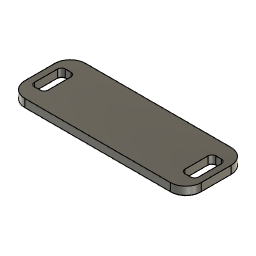
magnet spacer v1 (Autodesk Fusion 360 design; units mm, degrees)
Autodesk Fusion 360 part; units mm, degrees
sketch "Sketch1" plane through (0, 0, 0) normal (0, 0, 1) x (1, 0, 0)
  line L0 (4, 0) -> (41.72, 0)
  line L1 (45.72, 4) -> (45.72, 11.75)
  line L2 (41.72, 15.75) -> (4, 15.75)
  line L3 (0, 11.75) -> (0, 0)
  line L4 (0, 7.8501) -> (45.72, 7.875)
  line L5 (0, 15.75) -> (3.36, 15.75)
  line L6 (3.36, 15.75) -> (3.36, 0)
  line L7 (3.36, 0) -> (0, 0)
  line L8 (0, 4) -> (0, 15.75)
  line L9 (45.72, 15.75) -> (42.36, 15.75)
  line L10 (42.36, 15.75) -> (42.36, 0)
  line L11 (42.36, 0) -> (45.72, 0)
  line L12 (45.72, 0) -> (45.72, 15.75)
  line L13 (4.11, 11.875) -> (2.61, 11.875)
  line L14 (1.61, 10.875) -> (1.61, 4.875)
  line L15 (2.61, 3.875) -> (4.11, 3.875)
  line L16 (5.11, 4.875) -> (5.11, 10.875)
  line L17 (5.11, 11.875) -> (1.61, 3.875) construction
  line L18 (1.61, 11.875) -> (5.11, 3.875) construction
  line L19 (41.61, 11.875) -> (43.11, 11.875)
  line L20 (44.11, 10.875) -> (44.11, 4.875)
  line L21 (43.11, 3.875) -> (41.61, 3.875)
  line L22 (40.61, 4.875) -> (40.61, 10.875)
  line L23 (40.61, 11.875) -> (44.11, 3.875) construction
  line L24 (44.11, 11.875) -> (40.61, 3.875) construction
  arc A0 (5.11, 10.875) -> (4.11, 11.875) centre (4.11, 10.875) ccw
  arc A1 (2.61, 11.875) -> (1.61, 10.875) centre (2.61, 10.875) ccw
  arc A2 (1.61, 4.875) -> (2.61, 3.875) centre (2.61, 4.875) ccw
  arc A3 (4.11, 3.875) -> (5.11, 4.875) centre (4.11, 4.875) ccw
  arc A4 (41.61, 11.875) -> (40.61, 10.875) centre (41.61, 10.875) ccw
  arc A5 (40.61, 4.875) -> (41.61, 3.875) centre (41.61, 4.875) ccw
  arc A6 (43.11, 3.875) -> (44.11, 4.875) centre (43.11, 4.875) ccw
  arc A7 (44.11, 10.875) -> (43.11, 11.875) centre (43.11, 10.875) ccw
  arc A8 (45.72, 11.75) -> (41.72, 15.75) centre (41.72, 11.75) ccw
  arc A9 (0, 4) -> (4, 0) centre (4, 4) ccw
  arc A10 (4, 15.75) -> (0, 11.75) centre (4, 11.75) ccw
  arc A11 (41.72, 0) -> (45.72, 4) centre (41.72, 4) ccw
  point P0 (45.72, 0)
  point P1 (3.36, 7.875)
  point P2 (42.36, 7.875)
  dimension "d1" = 45.72
  dimension "d2" = 15.75
  dimension "d5" = 3.36
  dimension "d6" = 15.75
  dimension "d7" = 3.36
  dimension "d8" = 15.75
  dimension "d9" = 3.5
  dimension "d10" = 8
  dimension "d11" = 3.5
  dimension "d12" = 8
  dimension "d13" = 1
  dimension "d14" = 1
  dimension "d15" = 4
  dimension "d16" = 4
  constraint horizontal L0
  constraint vertical L1
  constraint horizontal L2
  constraint vertical L3
  constraint coincident L3.end L7.end
  constraint coincident L3 L4.start
  constraint horizontal L5
  constraint vertical L6
  constraint horizontal L7
  constraint vertical L8
  constraint horizontal L9
  constraint vertical L10
  constraint horizontal L11
  constraint vertical L12
  constraint horizontal L13
  constraint perpendicular L13 L14
  constraint parallel L13 L15
  constraint parallel L14 L16
  constraint coincident L17 P1
  constraint coincident L18 P1
  constraint midpoint L6 P1
  constraint horizontal L19
  constraint perpendicular L19 L20
  constraint parallel L19 L21
  constraint parallel L20 L22
  constraint coincident L23 P2
  constraint coincident L24 P2
  constraint midpoint L10 P2
  constraint coincident L17.start L13
  constraint coincident L17.start L16
  constraint tangent L13 A0
  constraint tangent L16 A0
  constraint coincident L18.start L13
  constraint coincident L18.start L14
  constraint tangent L13 A1
  constraint tangent L14 A1
  constraint equal A0 A1
  constraint coincident L17.end L14
  constraint coincident L17.end L15
  constraint tangent L14 A2
  constraint tangent L15 A2
  constraint equal A0 A2
  constraint coincident L18.end L15
  constraint coincident L18.end L16
  constraint tangent L15 A3
  constraint tangent L16 A3
  constraint equal A0 A3
  constraint coincident L23.start L19
  constraint coincident L23.start L22
  constraint tangent L19 A4
  constraint tangent L22 A4
  constraint equal A0 A4
  constraint coincident L24.end L22
  constraint coincident L24.end L21
  constraint tangent L22 A5
  constraint tangent L21 A5
  constraint equal A0 A5
  constraint coincident L23.end L21
  constraint coincident L23.end L20
  constraint tangent L21 A6
  constraint tangent L20 A6
  constraint equal A0 A6
  constraint coincident L24.start L20
  constraint coincident L24.start L19
  constraint tangent L20 A7
  constraint tangent L19 A7
  constraint coincident L1 L4.end
  constraint coincident L9.start L2
  constraint coincident L9.start L1
  constraint tangent L2 A8
  constraint tangent L1 A8
  constraint coincident L3.end L8
  constraint coincident L3.end L0
  constraint tangent L8 A9
  constraint tangent L0 A9
  constraint coincident L5.start L2
  constraint coincident L5.start L3
  constraint tangent L2 A10
  constraint tangent L3 A10
  constraint equal A9 A10
  constraint coincident P0 L0
  constraint coincident P0 L1
  constraint tangent L0 A11
  constraint tangent L1 A11
  constraint equal A9 A11
  measures "d1" distance of L3.end P0
  measures "d2" distance of L3.end L5.start
  measures "d5" distance of L5.start L5.end
  measures "d6" distance of L5.start L3.end
  measures "d7" distance of L9.start L9.end
  measures "d8" distance of L9.start P0
  measures "d9" distance of L17.end L18.end
  measures "d10" distance of L18.start L17.end
  measures "d11" distance of L23.end L24.end
  measures "d12" distance of L24.start L23.end
  measures "d13" radius of A0
  measures "d14" radius of A7
  measures "d15" radius of A8
  measures "d16" radius of A9
extrude "Extrude1" add sketch "Sketch1" along normal blind 2.25 contours L0 L4 L6 L10 L15 L16 L21 L22 A3 A5 A9 A11 | L3 L4 L6 L8 L14 L15 A2 A9 | L1 L4 L10 L12 L20 L21 A6 A11 | L3 L4 L6 L8 L13 L14 A1 A10 | L1 L4 L10 L12 L19 L20 A7 A8 | L2 L4 L6 L10 L13 L16 L19 L22 A0 A4 A8 A10
chamfer "Chamfer1" distance 0.2 angle 45 1 faces at (16.9298, 1.5311, 0)
